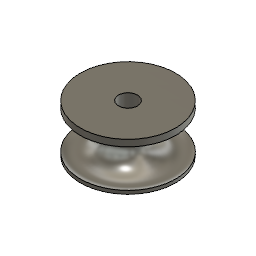
Spool (Autodesk Fusion 360 design; units mm, degrees)
part number: 2026-02-09-11-59-27-376
Autodesk Fusion 360 part; units mm, degrees
cylinder "CylinderPrimitive1" add diameter 32 height 1 placed x (1, 0, 0) y (0, 0, -1) z (0, 1, 0) at (0, 0, 0)
hole "Hole1" at (0, 1, 0) direction (0, -1, 0) diameter 6.35 depth 5 tip angle 118
extrude "Extrude1" add 1 faces at (11.6625, 1, 0.874) along direction (0, 1, 0) blind 15
move_body "Move1" bodies 1 to x (1, 0, 0) y (0, 1, 0) z (0, 0, 1) at (0, -7.5, 0)
torus "TorusPrimitive1" cut centre line diameter 26 section diameter 14 placed x (1, 0, 0) y (0, 0, -1) z (0, 1, 0) at (0, 0, 0)
